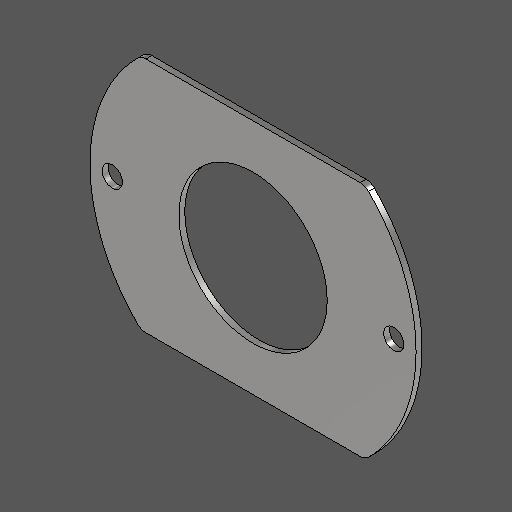
# Autodesk Inventor part: Plasma Box Slit
Saved by Autodesk Inventor 2025 (Build 290162000, 162)
## iProperties
Created: 2024-05-16
Part Number: Plasma Box Slit
Material: Stainless Steel
Document SubType Name: Modeling
Designer: KAA
Density: 8 g/cm^3
Appearance: Semi-Polished
Author: KAA
Autodesk Inventor part; units mm, degrees
ref_plane "YZ Plane" through (0, 0, 0) normal (1, 0, 0) x (0, 1, 0)
ref_plane "XZ Plane" through (0, 0, 0) normal (0, 1, 0) x (-1, 0, 0)
ref_plane "XY Plane" through (0, 0, 0) normal (0, 0, 1) x (1, 0, 0)
sketch "Sketch1" plane through (0, 0, 0) normal (0, 0, 1) x (1, 0, 0)
  circle A0 centre (0, 0) radius 12.5
  circle A1 centre (0, 0) radius 27.5
  dimension "d2" = 25
  dimension "d3" = 55
  constraints: 2 centre point, 2 coincident
  measures "d2" diameter of A0
  measures "d3" diameter of A1
extrude "Extrusion1" add sketch "Sketch1" along normal blind 1
sketch "Sketch2" plane through (0, 0, 1) normal (0, 0, 1) x (1, 0, 0)
  circle A0 centre (0, 0) radius 23.75 construction
  point P0 (23.75, 0)
  dimension "d4" = 47.5
  constraints: 2 horizontal alignment, 1 coincident, 2 other
hole "Hole1" at (23.75, 0, 1) direction (0, 0, -1) diameter 3.4 end through all
pattern_circular "Circular Pattern1" count 4 over 360 about axis through (0, 0, 0) along (0, 0, 1) of "Hole1"
sketch "Sketch3" plane through (0, 0, 1) normal (0, 0, 1) x (1, 0, 0)
  line L0 (-30, 30) -> (30, 30)
  line L1 (30, 30) -> (30, 20)
  line L2 (30, 20) -> (-30, 20)
  line L3 (-30, 20) -> (-30, 30)
  point P0 (0, 0)
  point P1 (0, 20)
  dimension "d15" = 20
  dimension "d16" = 60
  dimension "d17" = 10
  constraints: 8 end point, 2 parallel, 1 horizontal, 1 midpoint, 1 perpendicular, 1 vertical alignment
  measures "d15" distance from line of L2 point (0, 0)
  measures "d16" distance of L0.start L0.end
  measures "d17" distance of L0.end L1.end
extrude "Extrusion2" cut sketch "Sketch3" against normal through all
mirror "Mirror1" about plane through (0, 0, 0) normal (0, 1, 0) of "Extrusion2"
fillet "Fillet2" radius 2 4 edges at (-18.8746, 20, 0.5) (18.8746, 20, 0.5) (-18.8746, -20, 0.5) (18.8746, -20, 0.5)
body "Solid1"
